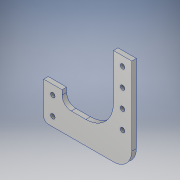
# Autodesk Inventor part: sidethrustalum
Saved by Autodesk Inventor 2017 (Build 210142000, 142)
## iProperties
Created: 2017-08-12
Part Number: sidethrustalum
Material: Aluminum 6061
Document SubType Name: Modeling
Designer: Kai
Density: 2.7 g/cm^3
Appearance: Aluminum - Flat
Author: Kai
Autodesk Inventor part; units mm, degrees
ref_plane "YZ Plane" through (0, 0, 0) normal (1, 0, 0) x (0, 1, 0)
ref_plane "XZ Plane" through (0, 0, 0) normal (0, 1, 0) x (-1, 0, 0)
ref_plane "XY Plane" through (0, 0, 0) normal (0, 0, 1) x (1, 0, 0)
sketch "Sketch1" plane through (0, 0, 0) normal (0, 0, 1) x (1, 0, 0)
  line L0 (0, 0) -> (0, 133.35)
  line L1 (0, 133.35) -> (-25.4, 133.35)
  line L2 (-25.4, 133.35) -> (-25.4, 69.85)
  line L3 (-63.5, 31.75) -> (-83.693, 31.75)
  line L4 (-96.393, 44.45) -> (-96.393, 50.8)
  line L5 (-96.393, 50.8) -> (-121.793, 50.8)
  line L6 (-121.793, 50.8) -> (-121.793, 0)
  line L7 (-121.793, 0) -> (0, 0)
  arc A0 (-96.393, 44.45) -> (-83.693, 31.75) centre (-83.693, 44.45) ccw
  arc A1 (-63.5, 31.75) -> (-25.4, 69.85) centre (-63.5, 69.85) ccw
  circle A2 centre (-12.7, 120.65) radius 3.1
  circle A3 centre (-12.7, 95.25) radius 3.1
  circle A4 centre (-12.7, 69.85) radius 3.1
  circle A5 centre (-12.7, 44.45) radius 3.1
  circle A6 centre (-109.093, 38.1) radius 3.1
  circle A7 centre (-109.093, 12.7) radius 3.1
  point P0 (-25.4, 31.75)
  point P1 (-96.393, 31.75)
  dimension "d0" = 133.35
  dimension "d1" = 25.4
  dimension "d2" = 101.6
  dimension "d3" = 70.993
  dimension "d4" = 19.05
  dimension "d5" = 25.4
  dimension "d6" = 12.7
  dimension "d7" = 38.1
  dimension "d8" = 6.2
  dimension "d9" = 12.7
  dimension "d10" = 12.7
  dimension "d13" = 25.4
  dimension "d18" = 6.2
  dimension "d19" = 12.7
  dimension "d20" = 12.7
  dimension "d21" = 6.2
  dimension "d22" = 25.4
  constraints: 16 end point, 8 centre point, 7 perpendicular, 4 point on circle, 4 point on line, 4 tangent, 2 vertical, 6 other
  measures "d0" distance of L0.start L0.end
  measures "d1" distance of L0.end L1.end
  measures "d2" distance of L1.end point (-25.4, 31.75)
  measures "d3" distance of point (-25.4, 31.75) point (-96.393, 31.75)
  measures "d4" distance of point (-96.393, 31.75) L4.end
  measures "d5" distance of L4.end L5.end
  measures "d6" radius of A0
  measures "d7" radius of A1
  measures "d8" diameter of A2
  measures "d9" distance from line of L1 A2.centre
  measures "d10" distance from line of L0 A2.centre
  measures "d13" distance of A2.centre A3.centre
  measures "d18" diameter of A6
  measures "d19" distance from line of A6.centre L5
  measures "d20" distance from line of L6 A6.centre
  measures "d21" diameter of A7
  measures "d22" distance of A7.centre A6.centre
extrude "Extrusion1" add sketch "Sketch1" along normal blind 6.35
fillet "Fillet1" radius 25.4 1 edges at (0, 0, 3.175)
fillet "Fillet2" radius 6.35 1 edges at (-121.793, 0, 3.175)
body "Solid1"
